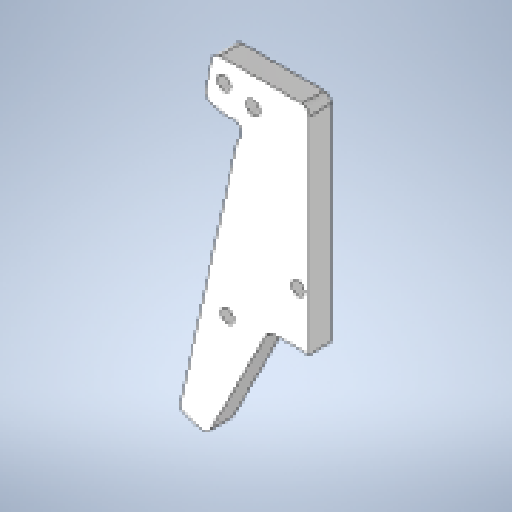
# Autodesk Inventor part: Uprights
Saved by Autodesk Inventor 2023.4 (Build 274418000, 418)
## iProperties
Created: 2024-02-11
Part Number: Uprights
Material: UHMW, White
Document SubType Name: Modeling
Designer: Nathan Cai
Density: 0.94 g/cm^3
Appearance: Smooth - White
Mass: 4.518 g
Surface Area: 30.6245 cm^2
Volume: 4.80639 cm^3
Author: Nathan Cai
Autodesk Inventor part; units mm, degrees
ref_plane "YZ Plane" through (0, 0, 0) normal (1, 0, 0) x (0, 1, 0)
ref_plane "XZ Plane" through (0, 0, 0) normal (0, 1, 0) x (-1, 0, 0)
ref_plane "XY Plane" through (0, 0, 0) normal (0, 0, 1) x (1, 0, 0)
sketch "Sketch1" plane through (0, 0, 0) normal (0, 0, 1) x (1, 0, 0)
  line L0 (0, 0) -> (0, 136.525) construction
  line L1 (-14.9636, 12.2907) -> (-42.8613, 18.4755) construction
  line L2 (-42.8613, 18.4755) -> (-36.5047, 47.1481) construction
  line L3 (-36.5047, 47.1481) -> (-8.607, 40.9633)
  line L4 (-8.607, 40.9633) -> (-14.9636, 12.2907) construction
  line L5 (-42.8613, 18.4755) -> (-8.607, 40.9633) construction
  line L6 (-36.5047, 47.1481) -> (-14.9636, 12.2907) construction
  circle A0 centre (-57.15, 12.7) radius 3.175 construction
  circle A1 centre (-57.15, 12.7) radius 6.35 construction
  line L7 (0, 0) -> (-57.847, 6.3884) construction
  line L8 (-62.7854, 15.6266) -> (0, 136.525) construction
  line L9 (-30.3052, 45.7737) -> (-40.6279, 28.5497) construction
  line L10 (-14.8065, 42.3377) -> (-12.7302, 22.3649) construction
  line L11 (-22.5559, 44.0557) -> (-28.9124, 15.3831) construction
  line L12 (0, 92.075) -> (-20.7006, 96.6642) construction
  line L13 (-38.5516, 8.5768) -> (-23.0529, 5.1408) construction
  line L14 (-23.0529, 5.1408) -> (-24.4273, -1.0586) construction
  line L15 (-24.4273, -1.0586) -> (-39.926, 2.3773) construction
  line L16 (-39.926, 2.3773) -> (-38.5516, 8.5768) construction
  line L17 (-38.5516, 8.5768) -> (-44.3299, 4.8956) construction
  line L18 (-23.0529, 5.1408) -> (-21.2746, 2.3495) construction
  line L19 (-8.607, 40.9633) -> (-36.5047, 47.1481) construction
  line L20 (-36.5047, 47.1481) -> (-35.4225, 52.0296) construction
  line L21 (-35.4225, 52.0296) -> (-7.5248, 45.8448) construction
  line L22 (-7.5248, 45.8448) -> (-8.607, 40.9633) construction
  line L23 (-56.4628, 15.7997) -> (-57.15, 12.7) construction
  line L24 (-57.15, 12.7) -> (-60.2497, 13.3872) construction
  line L25 (-30.8022, 6.8588) -> (-37.6742, -24.1386) construction
  line L26 (-35.0426, 50.076) -> (-8.6948, 44.2349)
  line L27 (-8.6948, 44.2349) -> (-7.664, 48.8845) construction
  line L28 (-7.664, 48.8845) -> (-34.0118, 54.7256) construction
  line L29 (-34.0118, 54.7256) -> (-35.0426, 50.076) construction
  line L30 (-34.5272, 52.4008) -> (-8.1794, 46.5597) construction
  circle A2 centre (-32.2024, 51.8854) radius 1.4732 construction
  circle A3 centre (-26.0029, 50.5111) radius 1.4732 construction
  circle A4 centre (-19.8034, 49.1367) radius 1.4732
  circle A5 centre (-13.6039, 47.7623) radius 1.4732
  circle A6 centre (-13.5364, 84.7398) radius 1.4732 construction
  line L31 (-57.15, 12.7) -> (-14.2841, 95.2417) construction
  line L32 (-34.4322, 56.4449) -> (0, 48.8115)
  circle A7 centre (-13.5364, 84.7398) radius 4.7625 construction
  line L33 (-4.7625, 49.8673) -> (-4.7625, 93.1308) construction
  line L34 (-29.6199, 55.378) -> (-16.3624, 80.9064) construction
  line L35 (-8.7753, 84.6261) -> (-4.7625, 83.7365) construction
  line L36 (-21.2746, 2.3495) -> (0, 2.3495) construction
  line L37 (0, 2.3495) -> (0, -0.8255) construction
  line L38 (0, -0.8255) -> (-21.2746, -0.8255) construction
  line L39 (-21.2746, -0.8255) -> (-21.2746, 2.3495) construction
  circle A8 centre (-15.875, 7.9375) radius 1.5875 construction
  line L40 (-15.875, 7.9375) -> (0, 7.9375)
  line L41 (0, 7.9375) -> (-21.2746, 2.3495) construction
  circle A9 centre (-15.875, 7.9375) radius 3.175 construction
  line L42 (-12.7, 7.9375) -> (-12.7, 4.6017) construction
  line L43 (-12.7, 7.9375) -> (0, 7.9375) construction
  line L44 (-21.0937, 46.9837) -> (-20.0629, 51.6333)
  line L45 (-15.6692, 45.7811) -> (-29.4131, -16.2137)
  line L46 (0, 66.675) -> (0, 7.9375)
  line L47 (-29.4131, -16.2137) -> (-23.2136, -17.5881)
  line L48 (-23.2136, -17.5881) -> (-8.7313, 7.9375)
  circle A10 centre (-15.875, 6.35) radius 1.4224
  line L49 (0, 13.4938) -> (-4.7625, 13.4938) construction
  line L50 (-4.7625, 13.4938) -> (-4.7625, 24.6063) construction
  line L51 (-4.7625, 24.6063) -> (0, 24.6063) construction
  line L52 (0, 24.6063) -> (0, 13.4938)
  line L53 (-4.7625, 19.05) -> (0, 19.05) construction
  circle A11 centre (-2.3813, 19.05) radius 1.4224
  line L54 (-23.9155, 8.5842) -> (-12.9204, 58.18)
  line L55 (-12.9204, 58.18) -> (-6.7209, 56.8056) construction
  line L56 (-6.7209, 56.8056) -> (-17.7161, 7.2098) construction
  line L57 (-17.7161, 7.2098) -> (-23.9155, 8.5842)
  line L58 (-15.875, 6.35) -> (-15.875, 7.9375) construction
  line L59 (-12.334, 1.5875) -> (-9.525, 1.5875)
  line L60 (-9.525, 1.5875) -> (-9.525, 7.9375)
  line L61 (-9.525, 7.9375) -> (-12.334, 7.9375)
  line L62 (-12.334, 7.9375) -> (-12.334, 1.5875) construction
  line L63 (-12.9204, 58.18) -> (-19.1199, 59.5544)
  line L64 (-19.1199, 59.5544) -> (-17.8882, 65.11)
  line L65 (-17.8882, 65.11) -> (0, 66.675)
  line L66 (-12.9204, 58.18) -> (-20.4943, 53.3549) construction
  arc A12 (-13.4063, 55.9882) -> (-15.1123, 58.6659) centre (-14.2593, 57.3271) ccw
  line L67 (-4.7625, 57.15) -> (0, 57.15) construction
  circle A13 centre (-2.3813, 57.15) radius 1.4224
  circle A14 centre (-2.3813, 63.5) radius 1.4224
  line L68 (-24.1057, 44.3993) -> (-22.0441, 53.6985)
  line L69 (-15.6692, 45.7811) -> (-19.4561, 43.3685) construction
  arc A15 (-16.2523, 43.1508) -> (-18.2994, 46.3642) centre (-17.2758, 44.7575) ccw
  line L70 (-22.0441, 53.6985) -> (0, 53.6985)
  line L71 (-16.3564, 42.6813) -> (-17.963, 41.6578) construction
  circle A16 centre (-17.963, 41.6578) radius 1.905
  point P0 (-25.7341, 29.7194)
  point P1 (-23.6144, 2.6079)
  point P2 (-39.4863, 4.3607)
  point P3 (-54.2234, 18.3354)
  point P4 (-14.2875, 7.9375)
  point P5 (-14.6033, 6.9872)
  point P6 (-11.9574, 7.9375)
  point P7 (-17.1467, 6.9872)
  point P8 (-15.6692, 45.7811)
  point P9 (-9.525, 6.5385)
  point P10 (-16.2523, 43.1508)
  point P11 (-18.9866, 43.2644)
  point P12 (-16.9395, 40.0511)
  dimension "d74" = 6.35
  dimension "d122" = 3.81
  dimension "d13" = 136.525
  dimension "d14" = 29.3687
  dimension "d15" = 28.575
  dimension "d16" = 12.5
  dimension "d17" = 6.35
  dimension "d19" = 57.15
  dimension "d22" = 12.7
  dimension "d23" = 7.9375
  dimension "d24" = 19.05
  dimension "d26" = 102.5
  dimension "d29" = 6.35
  dimension "d31" = 7.9375
  dimension "d34" = 5
  dimension "d35" = 26.9875
  dimension "d38" = 31.75
  dimension "d40" = 26.9875
  dimension "d41" = 4.7625
  dimension "d42" = 2.9464
  dimension "d43" = 2.3813
  dimension "d46" = 6.35
  dimension "d51" = 2.9464
  dimension "d52" = 79.7719
  dimension "d53" = 6.35
  dimension "d54" = 9.525
  dimension "d55" = 4.7625
  dimension "d56" = 4.7625
  dimension "d60" = 12.7
  dimension "d61" = 3.175
  dimension "d63" = 3.175
  dimension "d66" = 3.175
  dimension "d67" = 15.875
  dimension "d72" = 8.7312
  dimension "d73" = 7.9375
  dimension "d75" = 34.925
  dimension "d80" = 12.7
  dimension "d82" = 7.9375
  dimension "d83" = 63.5
  dimension "d84" = 66.675
  dimension "d85" = 6.35
  dimension "d86" = 92.075
  dimension "d87" = 2.8448
  dimension "d88" = 4.7625
  dimension "d89" = 11.1125
  dimension "d90" = 2.8448
  dimension "d91" = 19.05
  dimension "d92" = 6.35
  dimension "d93" = 50.8
  dimension "d94" = 25.4
  dimension "d95" = 8.7312
  dimension "d96" = 9.525
  dimension "d97" = 6.35
  dimension "d99" = 6.35
  dimension "d101" = 3.175
  dimension "d106" = 2.8448
  dimension "d107" = 57.15
  dimension "d110" = 6.35
  dimension "d119" = 85
  dimension "d120" = 3.175
  dimension "d121" = 3.81
  constraints: 144 end point, 50 point on line, 24 parallel, 21 perpendicular, 15 centre point, 14 point on circle, 11 coincident, 10 midpoint, 5 vertical, 3 horizontal, 2 collinear, 2 tangent, 1 horizontal alignment, 20 other
  measures "d13" distance of L0.start L0.end
  measures "d14" distance of L1.end L2.end
  measures "d15" distance between parallel lines of L4 L2
  measures "d16" angle of L0 L4
  measures "d17" diameter of A0
  measures "d19" distance from line of L0 A0.centre
  measures "d22" diameter of A1
  measures "d23" distance from line of L9.start L11
  measures "d24" distance from line of L9.end L3
  measures "d26" angle of L0 L12
  measures "d29" distance of L13.end L14.end
  measures "d31" distance between parallel lines of L14 L11
  measures "d34" distance of L2.end L20.end
  measures "d35" distance between parallel lines of L11 L23
  measures "d38" distance of L25.start L25.end
  measures "d40" distance between parallel lines of L27 L29
  measures "d41" distance between parallel lines of L26 L28
  measures "d42" diameter of A2
  measures "d43" distance from line of L29 A2.centre
  measures "d46" distance of A2.centre A3.centre
  measures "d51" diameter of A6
  measures "d52" distance from line of L13 A6.centre
  measures "d53" distance between parallel lines of L32 L26
  measures "d54" diameter of A7
  measures "d55" distance between parallel lines of L0 L33
  measures "d56" distance between parallel lines of L31 L34
  measures "d60" vertical distance of A0.centre L0.start
  measures "d61" distance between parallel lines of L3 L26
  measures "d63" distance between parallel lines of L36 L38
  measures "d66" diameter of A8
  measures "d67" distance from line of L0 A8.centre
  measures "d72" distance between parallel lines of L1 L13
  measures "d73" distance from line of L0.start L40
  measures "d75" vertical distance of point (0, 48.811) point (-4.763, 83.736)
  measures "d80" distance between parallel lines of L27 L44
  measures "d82" distance between parallel lines of L4 L45
  measures "d83" distance from line of L45.end L26
  measures "d84" distance of L0.start L46.start
  measures "d85" distance of L45.end L47.end
  measures "d86" distance of L0.start point (0, 92.075)
  measures "d87" diameter of A10
  measures "d88" distance of L50.end L51.end
  measures "d89" distance of L49.end L50.end
  measures "d90" diameter of A11
  measures "d91" distance from line of L0.start L53
  measures "d92" distance between parallel lines of L54 L56
  measures "d93" distance between parallel lines of L55 L57
  measures "d94" distance between parallel lines of L47 L57
  measures "d95" distance from line of L0 L48.end
  measures "d96" distance between parallel lines of L0 L60
  measures "d97" distance between parallel lines of L40 L59
  measures "d99" distance of L63.start L63.end
  measures "d101" diameter of A12
  measures "d106" diameter of A13
  measures "d107" distance from line of L0.start L67
  measures "d110" distance of A13.centre A14.centre
  measures "d119" angle of L0 L65
  measures "d120" distance from line of A4.centre L68
  measures "d121" diameter of A15
extrude "Extrusion1" add sketch "Sketch1" along normal blind 4.7625 contours L68 L26 L45 A16 L3 | L68 L32 L54 A15 L26 | L45 A15 L54 L32 L46 L40 L60 L48 L47 A16 | L70 L54 L32 | L45 A15 | A15 L26 | L54 L70 L46 L32 | L60 L40 L48
fillet "Fillet1" radius 1.5875 3 edges at (-29.4131, -16.2137, 2.3813) (-23.2136, -17.5881, 2.3813) (-8.7313, 7.9375, 2.3813)
fillet "Fillet4" radius 1.5875 5 edges at (-22.0441, 53.6985, 2.3813) (0, 53.6985, 2.3813) (-24.1057, 44.3993, 2.3813) (-18.9866, 43.2644, 2.3813) (-16.9395, 40.0511, 2.3813)
equation "\"d56\" = d55"
body "Solid1"
